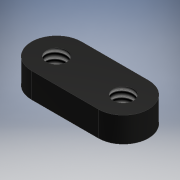
# Autodesk Inventor part: EPS_SwitchNut
Saved by Autodesk Inventor 2018 (Build 220112000, 112)
## iProperties
Created: 2018-05-30
Part Number: EPS_SwitchNut
Material: Aluminum 6061
Document SubType Name: Modeling
Designer: Bradley
Density: 2.7 g/cm^3
Appearance: Anodized - Dark Gray
Author: Bradley
Autodesk Inventor part; units mm, degrees
ref_plane "YZ Plane" through (0, 0, 0) normal (1, 0, 0) x (0, 1, 0)
ref_plane "XZ Plane" through (0, 0, 0) normal (0, 1, 0) x (-1, 0, 0)
ref_plane "XY Plane" through (0, 0, 0) normal (0, 0, 1) x (1, 0, 0)
sketch "Sketch1" plane through (0, 0, 0) normal (0, 0, 1) x (1, 0, 0)
  line L0 (-2, 0) -> (2, 0) construction
  line L1 (-2, -1.5) -> (2, -1.5)
  line L2 (2, 1.5) -> (-2, 1.5)
  arc A0 (-2, 1.5) -> (-2, -1.5) centre (-2, 0) ccw
  arc A1 (2, -1.5) -> (2, 1.5) centre (2, 0) ccw
  point P0 (0, 0)
  dimension "d1" = 3
  dimension "d11" = 4
  constraints: 8 end point, 4 point on circle, 4 tangent, 2 centre point, 1 horizontal, 1 midpoint, 1 parallel
  measures "d1" diameter of A1
  measures "d11" distance of L2.start L2.end
extrude "Extrusion1" add sketch "Sketch1" along normal mid plane 1.5
sketch "Sketch2" plane through (0, 0, 0.75) normal (0, 0, 1) x (1, 0, 0)
  line L0 (-2, -1.5) -> (2, -1.5) projected
  arc A0 (2, -1.5) -> (2, 1.5) centre (2, 0) ccw projected
  line L1 (2, 1.5) -> (-2, 1.5) projected
  arc A1 (-2, 1.5) -> (-2, -1.5) centre (-2, 0) ccw projected
  point P0 (0, 0)
  constraints: 2 coincident
hole "Hole1" at (-2, 0, 0.75) at (2, 0, 0.75) direction (0, 0, -1) diameter 1.221 end through all thread size "M1.6x0.35" class "6H" standard "ANSI Metric M Profile"
body "Solid1"
